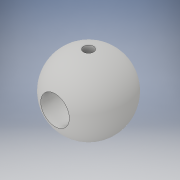
# Autodesk Inventor part: VS-008 (HANDLE BALL)
Saved by Autodesk Inventor 2017 (Build 210142000, 142)
## iProperties
Created: 2016-12-07
Part Number: VS-008 (HANDLE BALL)
Material: Generic
Document SubType Name: Modeling
Designer: OCCC
Density: 1 g/cm^3
Appearance: Default
Author: OCCC
Autodesk Inventor part; units mm, degrees
ref_plane "YZ Plane" through (0, 0, 0) normal (1, 0, 0) x (0, 1, 0)
sketch "Sketch1" plane through (0, 0, 0) normal (0, 1, 0) x (-1, 0, 0)
  line L0 (0, 0) -> (19.05, 0)
  arc A0 (19.05, 0) -> (0, 0) centre (9.525, 0) ccw
  dimension "d0" = 19.05
  constraints: 2 end point, 2 point on circle, 1 centre point, 1 horizontal, 1 midpoint
  measures "d0" distance of L0.start L0.end
revolve "Revolution1" add sketch "Sketch1" angle 360 about axis through (0, 0, 0) along (-1, 0, 0)
ref_plane "Work Plane1" through (-9.525, 9.525, 0) normal (0, 1, 0) x (-1, 0, 0)
ref_plane "Work Plane2" through (0, 0, 9.525) normal (0, 0, 1) x (1, 0, 0)
sketch "Sketch5" plane through (-9.525, 9.525, 0) normal (0, 1, 0) x (-1, 0, 0)
  circle A0 centre (0, 0) radius 1.3208
  point P0 (-9.525, 0)
  dimension "d19" = 2.6416
  dimension "d20" = 9.525
  constraints: 1 centre point, 1 horizontal alignment
  measures "d19" diameter of A0
  measures "d20" distance of A0.centre point (-9.525, 0)
extrude "Extrusion1" cut sketch "Sketch5" against normal through all
sketch "Sketch6" plane through (0, 0, 9.525) normal (0, 0, 1) x (1, 0, 0)
  circle A0 centre (-9.525, 0) radius 3.7465
  point P0 (0, 0)
  dimension "d23" = 9.525
  dimension "d24" = 7.493
  constraints: 1 centre point, 1 horizontal alignment
  measures "d23" distance of point (0, 0) A0.centre
  measures "d24" diameter of A0
extrude "Extrusion2" cut sketch "Sketch6" against normal blind 12.7
body "Solid1"
